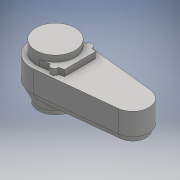
# Autodesk Inventor part: 1
Saved by Autodesk Inventor 2016 (Build 200138000, 138)
## iProperties
Created: 2015-12-17
Part Number: 1
Material: Generic
Document SubType Name: Modeling
Designer: ajshort
Density: 1 g/cm^3
Appearance: Default
Author: ajshort
Autodesk Inventor part; units mm, degrees
ref_plane "YZ Plane" through (0, 0, 0) normal (1, 0, 0) x (0, 1, 0)
sketch "Sketch1" plane through (0, 0, 0) normal (0, 0, 1) x (1, 0, 0)
  circle A0 centre (0, 0) radius 94
  dimension "d0" = 188
  constraints: 1 centre point, 1 coincident
  measures "d0" diameter of A0
extrude "Extrusion1" add sketch "Sketch1" along normal blind 20.292
ref_plane "Work Plane1" through (0, 0, 105) normal (0, 0, -1) x (-1, 0, 0)
sketch "Sketch2" plane through (0, 0, 105) normal (0, 0, -1) x (-1, 0, 0)
  circle A0 centre (0, 0) radius 133.5
  dimension "d4" = 267
  constraints: 1 centre point, 1 coincident
  measures "d4" diameter of A0
loft "Loft1" add profiles "Sketch2" section 2 edges at (-94, 0, 20.292)
sketch "Sketch3" plane through (0, 0, 105) normal (0, 0, 1) x (1, 0, 0)
  circle A0 centre (0, 0) radius 133.5 construction
  circle A1 centre (425, 0) radius 89 construction
  line L0 (13.9782, 132.7662) -> (434.3188, 88.5108)
  circle A2 centre (0, 0) radius 133.5 projected
  line L1 (13.9782, -132.7662) -> (434.3188, -88.5108)
  arc A3 (13.9782, 132.7662) -> (13.9782, -132.7662) centre (0, 0) ccw
  arc A4 (434.3188, -88.5108) -> (434.3188, 88.5108) centre (425, 0) ccw
  dimension "d9" = 178
  dimension "d10" = 425
  constraints: 8 point on circle, 4 end point, 3 centre point, 2 coincident, 2 tangent, 1 equal length, 1 horizontal alignment, 1 vertical alignment
  measures "d9" diameter of A1
  measures "d10" distance of A1.centre point (0, 0)
extrude "Extrusion2" add sketch "Sketch3" along normal blind 121
ref_plane "Work Plane2" through (0, 0, 74) normal (0, 0, -1) x (-1, 0, 0)
sketch "Sketch4" plane through (0, 0, 74) normal (0, 0, -1) x (-1, 0, 0)
  arc A0 (-434.3188, 88.5108) -> (-434.3188, -88.5108) centre (-425, 0) ccw construction
  circle A1 centre (-425, 0) radius 74.544 construction
  circle A2 centre (0, 0) radius 119.044 construction
  line L0 (-12.4646, -118.3896) -> (-432.8052, -74.1342)
  line L1 (-12.4646, 118.3896) -> (-432.8052, 74.1342)
  line L2 (-13.9782, -132.7662) -> (-434.3188, -88.5108) projected
  line L3 (-434.3188, 88.5108) -> (-13.9782, 132.7662) projected
  arc A3 (-12.4646, -118.3896) -> (-12.4646, 118.3896) centre (0, 0) ccw
  arc A4 (-432.8052, 74.1342) -> (-432.8052, -74.1342) centre (-425, 0) ccw
  dimension "d14" = 149.088
  dimension "d15" = 238.088
  constraints: 8 point on circle, 4 centre point, 4 coincident, 4 end point, 2 parallel, 2 tangent
  measures "d14" diameter of A1
  measures "d15" diameter of A2
loft "Loft2" add profiles "Sketch4" section 2 edges at (133.5, 0, 105) (224.1485, 110.6385, 105) (514, 0, 105) (224.1485, -110.6385, 105)
sketch "Sketch7" plane through (0, 0, 226) normal (0, 0, 1) x (1, 0, 0)
  circle A0 centre (0, 0) radius 108 construction
  line L0 (135, 85.862) -> (135, -85.862)
  line L1 (135, -85.862) -> (135, 85.862) construction
  line L2 (18.7539, 106.3592) -> (135, 85.862) construction
  line L3 (135, -85.862) -> (18.7539, -106.3592) construction
  circle A1 centre (89, 93.973) radius 20 construction
  circle A2 centre (89, -93.973) radius 20 construction
  line L4 (135, 85.862) -> (108.6962, 90.5001)
  line L5 (135, -85.862) -> (108.6962, -90.5001)
  arc A3 (69.3038, -97.446) -> (108.6962, -90.5001) centre (89, -93.973) ccw
  arc A4 (108.6962, 90.5001) -> (69.3038, 97.446) centre (89, 93.973) ccw
  line L6 (69.3038, 97.446) -> (18.7539, 106.3592)
  line L7 (69.3038, -97.446) -> (18.7539, -106.3592)
  arc A5 (18.7539, 106.3592) -> (18.7539, -106.3592) centre (0, 0) ccw
  point P0 (135, 0)
  dimension "d33" = 40
  dimension "d30" = 216
  dimension "d31" = 171.724
  dimension "d32" = 135
  dimension "d34" = 89
  constraints: 16 end point, 8 point on circle, 4 centre point, 4 coincident, 4 point on line, 4 tangent, 2 collinear, 1 horizontal alignment, 1 midpoint, 1 vertical, 1 vertical alignment, 7 other
  measures "d30" diameter of A0
  measures "d31" distance of L0.start L0.end
  measures "d32" distance from line of point (0, 0) L0
  measures "d34" horizontal distance of point (0, 0) point (89, -93.973)
extrude "Extrusion5" add sketch "Sketch7" along normal blind 34.5
sketch "Sketch8" plane through (0, 0, 260.5) normal (0, 0, 1) x (1, 0, 0)
  circle A0 centre (0, 0) radius 108
  arc A1 (18.7539, 106.3592) -> (18.7539, -106.3592) centre (0, 0) ccw construction
  point P0 (-108, 0)
  constraints: 1 coincident, 1 horizontal alignment, 1 point on circle, 2 other
extrude "Extrusion6" add sketch "Sketch8" along normal blind 34.5
body "Solid1"
